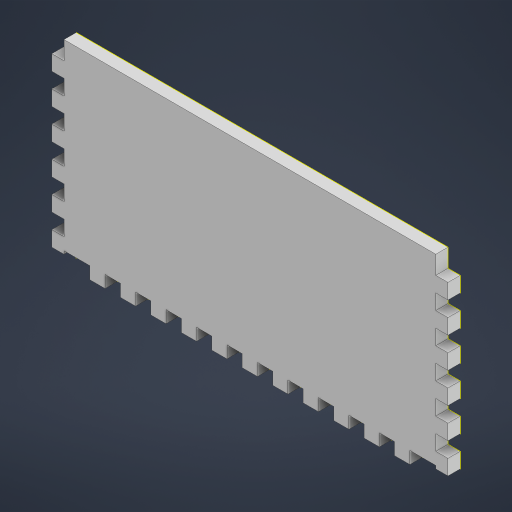
# Autodesk Inventor part: BackWand
Saved by Autodesk Inventor 2023 (Build 270158030, 158C)
## iProperties
Created: 2022-06-21
Part Number: BackWand
Material: Generic
Document SubType Name: Modeling
Designer: Simon
Density: 1 g/cm^3
Appearance: Default
Author: Simon
Autodesk Inventor part; units mm, degrees
ref_plane "YZ Plane" through (0, 0, 0) normal (1, 0, 0) x (0, 1, 0)
ref_plane "XZ Plane" through (0, 0, 0) normal (0, 1, 0) x (-1, 0, 0)
ref_plane "XY Plane" through (0, 0, 0) normal (0, 0, 1) x (1, 0, 0)
sketch "Sketch1" plane through (0, 0, 0) normal (0, 0, 1) x (1, 0, 0)
  line L0 (0, 3) -> (-4, 3)
  line L1 (0, 0) -> (0, 4)
  line L2 (8.5, 4) -> (0, 4)
  line L3 (8.5, 4) -> (8.5, 0)
  line L4 (13.5, 0) -> (8.5, 0)
  line L5 (13.5, 0) -> (13.5, 4)
  line L6 (18.5, 4) -> (13.5, 4)
  line L7 (18.5, 4) -> (18.5, 0)
  line L8 (23.5, 0) -> (18.5, 0)
  line L9 (23.5, 0) -> (23.5, 4)
  line L10 (28.5, 4) -> (23.5, 4)
  line L11 (28.5, 4) -> (28.5, 0)
  line L12 (33.5, 0) -> (28.5, 0)
  line L13 (33.5, 0) -> (33.5, 4)
  line L14 (38.5, 4) -> (33.5, 4)
  line L15 (38.5, 4) -> (38.5, 0)
  line L16 (43.5, 0) -> (38.5, 0)
  line L17 (43.5, 0) -> (43.5, 4)
  line L18 (48.5, 4) -> (43.5, 4)
  line L19 (48.5, 4) -> (48.5, 0)
  line L20 (53.5, 0) -> (48.5, 0)
  line L21 (53.5, 0) -> (53.5, 4)
  line L22 (58.5, 4) -> (53.5, 4)
  line L23 (58.5, 4) -> (58.5, 0)
  line L24 (63.5, 0) -> (58.5, 0)
  line L25 (63.5, 0) -> (63.5, 4)
  line L26 (68.5, 4) -> (63.5, 4)
  line L27 (68.5, 4) -> (68.5, 0)
  line L28 (73.5, 0) -> (68.5, 0)
  line L29 (73.5, 0) -> (73.5, 4)
  line L30 (78.5, 4) -> (73.5, 4)
  line L31 (83.5, 0) -> (78.5, 0)
  line L32 (78.5, 4) -> (78.5, 0)
  line L33 (83.5, 0) -> (83.5, 4)
  line L34 (88.5, 4) -> (83.5, 4)
  line L35 (88.5, 4) -> (88.5, 0)
  line L36 (93.5, 0) -> (88.5, 0)
  line L37 (93.5, 0) -> (93.5, 4)
  line L38 (98.5, 4) -> (93.5, 4)
  line L39 (98.5, 4) -> (98.5, 0)
  line L40 (103.5, 0) -> (98.5, 0)
  line L41 (103.5, 0) -> (103.5, 4)
  line L42 (108.5, 4) -> (103.5, 4)
  line L43 (108.5, 4) -> (108.5, 0)
  line L44 (113.5, 0) -> (108.5, 0)
  line L45 (113.5, 0) -> (113.5, 4)
  line L46 (122, 4) -> (113.5, 4)
  line L47 (126, 3) -> (122, 3)
  line L48 (122, 0) -> (122, 4)
  line L49 (126, 8) -> (126, 3)
  line L50 (126, 8) -> (122, 8)
  line L51 (122, 8) -> (122, 13)
  line L52 (126, 13) -> (122, 13)
  line L53 (126, 18) -> (126, 13)
  line L54 (126, 18) -> (122, 18)
  line L55 (122, 18) -> (122, 23)
  line L56 (126, 23) -> (122, 23)
  line L57 (126, 28) -> (126, 23)
  line L58 (126, 28) -> (122, 28)
  line L59 (122, 28) -> (122, 33)
  line L60 (126, 33) -> (122, 33)
  line L61 (126, 38) -> (126, 33)
  line L62 (126, 38) -> (122, 38)
  line L63 (122, 38) -> (122, 43)
  line L64 (126, 43) -> (122, 43)
  line L65 (126, 48) -> (126, 43)
  line L66 (126, 48) -> (122, 48)
  line L67 (122, 48) -> (122, 53)
  line L68 (126, 53) -> (122, 53)
  line L69 (126, 58) -> (126, 53)
  line L70 (126, 58) -> (122, 58)
  line L71 (122, 58) -> (122, 68)
  line L72 (-4, 8) -> (-4, 3)
  line L73 (0, 8) -> (-4, 8)
  line L74 (0, 13) -> (0, 8)
  line L75 (0, 13) -> (-4, 13)
  line L76 (-4, 18) -> (-4, 13)
  line L77 (0, 18) -> (-4, 18)
  line L78 (0, 23) -> (0, 18)
  line L79 (0, 23) -> (-4, 23)
  line L80 (-4, 28) -> (-4, 23)
  line L81 (0, 28) -> (-4, 28)
  line L82 (0, 33) -> (0, 28)
  line L83 (-4, 33) -> (0, 33)
  line L84 (-4, 38) -> (-4, 33)
  line L85 (0, 38) -> (-4, 38)
  line L86 (0, 43) -> (0, 38)
  line L87 (0, 43) -> (-4, 43)
  line L88 (-4, 48) -> (-4, 43)
  line L89 (0, 48) -> (-4, 48)
  line L90 (0, 53) -> (0, 48)
  line L91 (-4, 53) -> (0, 53)
  line L92 (-4, 58) -> (-4, 53)
  line L93 (0, 58) -> (-4, 58)
  line L94 (0, 68) -> (0, 58)
  line L95 (0, 64) -> (122, 64)
  point P0 (0, 0)
  constraints: 192 end point, 1 horizontal
extrude "Extrusion1" add sketch "Sketch1" along normal blind 4
sketch "Sketch2" plane through (0, 0, 0) normal (0, 0, -1) x (-1, 0, 0)
  line L0 (-8.5, 4) -> (-8.5, 0) projected
  line L1 (0, 4) -> (-8.5, 4) projected
  line L2 (0, 3) -> (0, 4) projected
  line L3 (4, 3) -> (0, 3) projected
  line L4 (4, 8) -> (4, 3) projected
  line L5 (0, 8) -> (4, 8) projected
  line L6 (0, 13) -> (0, 8) projected
  line L7 (4, 13) -> (0, 13) projected
  line L8 (4, 18) -> (4, 13) projected
  line L9 (0, 18) -> (4, 18) projected
  line L10 (0, 23) -> (0, 18) projected
  line L11 (4, 23) -> (0, 23) projected
  line L12 (4, 28) -> (4, 23) projected
  line L13 (0, 28) -> (4, 28) projected
  line L14 (0, 33) -> (0, 28) projected
  line L15 (4, 33) -> (0, 33) projected
  line L16 (4, 38) -> (4, 33) projected
  line L17 (0, 38) -> (4, 38) projected
  line L18 (0, 43) -> (0, 38) projected
  line L19 (4, 43) -> (0, 43) projected
  line L20 (4, 48) -> (4, 43) projected
  line L21 (0, 48) -> (4, 48) projected
  line L22 (0, 53) -> (0, 48) projected
  line L23 (4, 53) -> (0, 53) projected
  line L24 (4, 58) -> (4, 53) projected
  line L25 (0, 58) -> (4, 58) projected
  line L26 (0, 64) -> (0, 58) projected
  line L27 (-122, 64) -> (0, 64) projected
  line L28 (-122, 58) -> (-122, 64) projected
  line L29 (-126, 58) -> (-122, 58) projected
  line L30 (-126, 53) -> (-126, 58) projected
  line L31 (-122, 53) -> (-126, 53) projected
  line L32 (-122, 48) -> (-122, 53) projected
  line L33 (-126, 48) -> (-122, 48) projected
  line L34 (-126, 43) -> (-126, 48) projected
  line L35 (-122, 43) -> (-126, 43) projected
  line L36 (-122, 38) -> (-122, 43) projected
  line L37 (-126, 38) -> (-122, 38) projected
  line L38 (-126, 33) -> (-126, 38) projected
  line L39 (-122, 33) -> (-126, 33) projected
  line L40 (-122, 28) -> (-122, 33) projected
  line L41 (-126, 28) -> (-122, 28) projected
  line L42 (-126, 23) -> (-126, 28) projected
  line L43 (-122, 23) -> (-126, 23) projected
  line L44 (-122, 18) -> (-122, 23) projected
  line L45 (-126, 18) -> (-122, 18) projected
  line L46 (-126, 13) -> (-126, 18) projected
  line L47 (-122, 13) -> (-126, 13) projected
  line L48 (-122, 8) -> (-122, 13) projected
  line L49 (-126, 8) -> (-122, 8) projected
  line L50 (-126, 3) -> (-126, 8) projected
  line L51 (-122, 3) -> (-126, 3) projected
  line L52 (-122, 4) -> (-122, 3) projected
  line L53 (-113.5, 4) -> (-122, 4) projected
  line L54 (-113.5, 0) -> (-113.5, 4) projected
  line L55 (-108.5, 0) -> (-113.5, 0) projected
  line L56 (-108.5, 4) -> (-108.5, 0) projected
  line L57 (-103.5, 4) -> (-108.5, 4) projected
  line L58 (-103.5, 0) -> (-103.5, 4) projected
  line L59 (-98.5, 0) -> (-103.5, 0) projected
  line L60 (-98.5, 4) -> (-98.5, 0) projected
  line L61 (-93.5, 4) -> (-98.5, 4) projected
  line L62 (-93.5, 0) -> (-93.5, 4) projected
  line L63 (-88.5, 0) -> (-93.5, 0) projected
  line L64 (-88.5, 4) -> (-88.5, 0) projected
  line L65 (-83.5, 4) -> (-88.5, 4) projected
  line L66 (-83.5, 0) -> (-83.5, 4) projected
  line L67 (-78.5, 0) -> (-83.5, 0) projected
  line L68 (-78.5, 4) -> (-78.5, 0) projected
  line L69 (-73.5, 4) -> (-78.5, 4) projected
  line L70 (-73.5, 0) -> (-73.5, 4) projected
  line L71 (-68.5, 0) -> (-73.5, 0) projected
  line L72 (-68.5, 4) -> (-68.5, 0) projected
  line L73 (-63.5, 4) -> (-68.5, 4) projected
  line L74 (-63.5, 0) -> (-63.5, 4) projected
  line L75 (-58.5, 0) -> (-63.5, 0) projected
  line L76 (-58.5, 4) -> (-58.5, 0) projected
  line L77 (-53.5, 4) -> (-58.5, 4) projected
  line L78 (-53.5, 0) -> (-53.5, 4) projected
  line L79 (-48.5, 0) -> (-53.5, 0) projected
  line L80 (-48.5, 4) -> (-48.5, 0) projected
  line L81 (-43.5, 4) -> (-48.5, 4) projected
  line L82 (-43.5, 0) -> (-43.5, 4) projected
  line L83 (-38.5, 0) -> (-43.5, 0) projected
  line L84 (-38.5, 4) -> (-38.5, 0) projected
  line L85 (-33.5, 4) -> (-38.5, 4) projected
  line L86 (-33.5, 0) -> (-33.5, 4) projected
  line L87 (-28.5, 0) -> (-33.5, 0) projected
  line L88 (-28.5, 4) -> (-28.5, 0) projected
  line L89 (-23.5, 4) -> (-28.5, 4) projected
  line L90 (-23.5, 0) -> (-23.5, 4) projected
  line L91 (-18.5, 0) -> (-23.5, 0) projected
  line L92 (-18.5, 4) -> (-18.5, 0) projected
  line L93 (-13.5, 4) -> (-18.5, 4) projected
  line L94 (-13.5, 0) -> (-13.5, 4) projected
  line L95 (-8.5, 0) -> (-13.5, 0) projected
  point P0 (0, 0)
body "Solid1"
